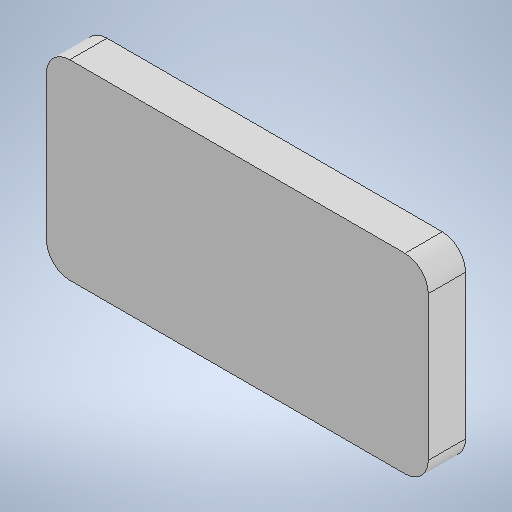
# Autodesk Inventor part: servo mout platform
Saved by Autodesk Inventor 2025.1 (Build 291241000, 241)
## iProperties
Created: 2025-03-10
Part Number: servo mout platform
Material: Generic
Document SubType Name: Modeling
Designer: vessy
Density: 1 g/cm^3
Appearance: Default
Author: vessy
Autodesk Inventor part; units mm, degrees
ref_plane "YZ Plane" through (0, 0, 0) normal (1, 0, 0) x (0, 1, 0)
ref_plane "XZ Plane" through (0, 0, 0) normal (0, 1, 0) x (-1, 0, 0)
ref_plane "XY Plane" through (0, 0, 0) normal (0, 0, 1) x (1, 0, 0)
sketch "Sketch1" plane through (0, 0, 0) normal (0, 0, 1) x (1, 0, 0)
  line L0 (0, 0) -> (52, 0)
  line L1 (52, 0) -> (52, -26)
  line L2 (52, -26) -> (0, -26)
  line L3 (0, -26) -> (0, 0)
  dimension "d0" = 52
  dimension "d1" = 26
  constraints: 8 end point, 2 parallel, 1 horizontal, 1 perpendicular
  measures "d0" distance of L0.start L0.end
  measures "d1" distance of L2.end L0.start
extrude "Extrusion1" add sketch "Sketch1" along normal blind 5.08
fillet "Fillet1" radius 3.175 4 edges at (52, 0, 2.54) (0, 0, 2.54) (52, -26, 2.54) (0, -26, 2.54)
body "Solid1"
